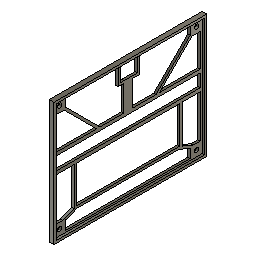
Platine_220 v2 (Autodesk Fusion 360 design; units mm, degrees)
Autodesk Fusion 360 part; units mm, degrees
note: some values were not read from the file. Set by a fixed rule: the direction of a hole.
(part 1 of 10)
sketch "Skizze1" plane through (0, 0, 0) normal (1, 0, 0) x (0, 1, 0)
  line L0 (7.62, 80.01) -> (3.81, 76.2)
  line L1 (99.695, 6.985) -> (99.695, 73.025)
  line L2 (0, 72.39) -> (0, 7.62)
  line L3 (92.71, 80.01) -> (7.62, 80.01)
  line L4 (7.62, 0) -> (92.71, 0)
  line L5 (99.695, 73.025) -> (92.71, 80.01)
  line L6 (3.81, 76.2) -> (0, 72.39)
  line L7 (0, 7.62) -> (7.62, 0)
  line L8 (92.71, 0) -> (99.695, 6.985)
  line L9 (5.5681, 3.81) -> (5.4821, 4.3533)
  line L10 (4.8434, 74.7776) -> (5.2324, 75.1666)
  line L11 (95.9767, 74.5279) -> (96.52, 74.4419)
  line L12 (95.0976, 75.1666) -> (95.4866, 74.7776)
  line L13 (95.9767, 5.4821) -> (95.4866, 5.2324)
  line L14 (5.4821, 4.3533) -> (5.2324, 4.8434)
  line L15 (5.123, 2.6407) -> (5.3653, 2.9903)
  line L16 (97.6893, 74.887) -> (99.5934, 72.9829)
  line L17 (3.3878, 74.4933) -> (3.81, 74.4419)
  line L18 (5.3653, 77.0197) -> (5.123, 77.3693)
  line L19 (94.9647, 77.0197) -> (94.8133, 76.6222)
  line L20 (2.9903, 5.3653) -> (2.6407, 5.123)
  line L21 (99.5934, 7.0271) -> (97.6893, 5.123)
  line L22 (96.52, 74.4419) -> (96.9422, 74.4933)
  line L23 (97.3397, 5.3653) -> (96.9422, 5.5167)
  line L24 (2.6407, 5.123) -> (0.3581, 7.4055)
  line L25 (4.8434, 5.2324) -> (4.3533, 5.4821)
  line L26 (7.4055, 0.3581) -> (5.123, 2.6407)
  line L27 (2.6407, 74.887) -> (2.9903, 74.6447)
  line L28 (0.3581, 7.4055) -> (0.3581, 72.6045)
  line L29 (3.81, 5.5681) -> (3.3878, 5.5167)
  line L30 (94.8133, 76.6222) -> (94.7619, 76.2)
  line L31 (4.3533, 5.4821) -> (3.81, 5.5681)
  line L32 (5.2324, 4.8434) -> (4.8434, 5.2324)
  line L33 (95.4866, 74.7776) -> (95.9767, 74.5279)
  line L34 (97.3397, 74.6447) -> (97.6893, 74.887)
  line L35 (94.8479, 75.6567) -> (95.0976, 75.1666)
  line L36 (94.7619, 3.81) -> (94.8133, 3.3878)
  line L37 (94.9647, 2.9903) -> (95.207, 2.6407)
  line L38 (5.5681, 76.2) -> (5.5167, 76.6222)
  line L39 (2.9903, 74.6447) -> (3.3878, 74.4933)
  line L40 (95.0976, 4.8434) -> (94.8479, 4.3533)
  line L41 (5.4821, 75.6567) -> (5.5681, 76.2)
  line L42 (96.9422, 5.5167) -> (96.52, 5.5681)
  line L43 (94.8133, 3.3878) -> (94.9647, 2.9903)
  line L44 (95.207, 2.6407) -> (92.9245, 0.3581)
  line L45 (94.8479, 4.3533) -> (94.7619, 3.81)
  line L46 (5.123, 77.3693) -> (7.3955, 79.6419)
  line L47 (94.7619, 76.2) -> (94.8479, 75.6567)
  line L48 (92.9245, 0.3581) -> (7.4055, 0.3581)
  line L49 (96.52, 5.5681) -> (95.9767, 5.4821)
  line L50 (97.6893, 5.123) -> (97.3397, 5.3653)
  line L51 (95.4866, 5.2324) -> (95.0976, 4.8434)
  line L52 (99.5934, 72.9829) -> (99.5934, 7.0271)
  line L53 (95.207, 77.3693) -> (94.9647, 77.0197)
  line L54 (4.3533, 74.5279) -> (4.8434, 74.7776)
  line L55 (0.3581, 72.6045) -> (2.6407, 74.887)
  line L56 (3.81, 74.4419) -> (4.3533, 74.5279)
  line L57 (7.3955, 79.6419) -> (92.9345, 79.6419)
  line L58 (5.5167, 76.6222) -> (5.3653, 77.0197)
  line L59 (96.9422, 74.4933) -> (97.3397, 74.6447)
  line L60 (92.9345, 79.6419) -> (95.207, 77.3693)
  line L61 (5.2324, 75.1666) -> (5.4821, 75.6567)
  line L62 (3.3878, 5.5167) -> (2.9903, 5.3653)
  line L63 (5.3653, 2.9903) -> (5.5167, 3.3878)
  line L64 (5.5167, 3.3878) -> (5.5681, 3.81)
  line L65 (66.3187, 30.0127) -> (66.3964, 29.8966)
  line L66 (71.048, 33.3571) -> (71.048, 33.3571)
  line L67 (67.6402, 29.4615) -> (67.6402, 29.4615)
  line L68 (67.6402, 29.4615) -> (67.7773, 29.4887)
  line L69 (72.5965, 32.2321) -> (72.3652, 32.686)
  line L70 (72.5965, 31.2259) -> (72.6761, 31.729)
  line L71 (71.5511, 33.2775) -> (71.048, 33.3571)
  line L72 (66.9595, 32.2321) -> (66.8799, 31.729)
  line L73 (66.8055, 31.4532) -> (66.7266, 31.3936)
  line L74 (68.508, 33.3571) -> (68.508, 33.3571)
  line L75 (66.8799, 31.729) -> (66.8843, 31.6087)
  line L76 (66.7266, 29.5664) -> (66.7266, 29.5664)
  line L77 (66.7266, 31.3936) -> (66.3964, 31.0634)
  line L78 (72.3652, 30.772) -> (72.5965, 31.2259)
  line L79 (66.3964, 31.0634) -> (66.3187, 30.9473)
  line L80 (66.3187, 30.9473) -> (66.2915, 30.8102)
  line L81 (66.3964, 29.8966) -> (66.3964, 29.8966)
  line L82 (66.2915, 30.1498) -> (66.3187, 30.0127)
  line L83 (68.2934, 29.995) -> (68.3264, 30.111)
  line L84 (66.8976, 31.489) -> (66.8055, 31.4532)
  line L85 (72.005, 33.0462) -> (71.5511, 33.2775)
  line L86 (66.8843, 31.6087) -> (66.8976, 31.489)
  line L87 (68.4171, 30.1034) -> (68.508, 30.1009)
  line L88 (66.2915, 30.8102) -> (66.2915, 30.8102)
  line L89 (71.048, 30.1009) -> (71.5511, 30.1805)
  line L90 (72.3652, 32.686) -> (72.005, 33.0462)
  line L91 (67.8934, 29.5664) -> (68.2236, 29.8966)
  line L92 (66.2915, 30.1498) -> (66.2915, 30.1498)
  line L93 (67.8934, 29.5664) -> (67.8934, 29.5664)
  line L94 (68.2236, 29.8966) -> (68.2236, 29.8966)
  line L95 (67.551, 33.0462) -> (67.1908, 32.686)
  line L96 (68.508, 30.1009) -> (68.508, 30.1009)
  line L97 (71.048, 30.1009) -> (71.048, 30.1009)
  line L98 (66.2915, 30.8102) -> (66.2915, 30.1498)
  line L99 (66.3964, 31.0634) -> (66.3964, 31.0634)
  line L100 (68.508, 33.3571) -> (68.0049, 33.2775)
  line L101 (67.1908, 32.686) -> (66.9595, 32.2321)
  line L102 (66.7266, 31.3936) -> (66.7266, 31.3936)
  line L103 (71.048, 33.3571) -> (68.508, 33.3571)
  line L104 (66.7266, 29.5664) -> (66.8427, 29.4887)
  line L105 (71.5511, 30.1805) -> (72.005, 30.4118)
  line L106 (72.005, 30.4118) -> (72.3652, 30.772)
  line L107 (66.3964, 29.8966) -> (66.7266, 29.5664)
  line L108 (67.7773, 29.4887) -> (67.8934, 29.5664)
  line L109 (72.6761, 31.729) -> (72.5965, 32.2321)
  line L110 (66.9798, 29.4615) -> (66.9798, 29.4615)
  line L111 (68.2236, 29.8966) -> (68.2934, 29.995)
  line L112 (66.9798, 29.4615) -> (67.6402, 29.4615)
  line L113 (68.3264, 30.111) -> (68.4171, 30.1034)
  line L114 (66.8427, 29.4887) -> (66.9798, 29.4615)
  line L115 (68.508, 30.1009) -> (71.048, 30.1009)
  line L116 (68.0049, 33.2775) -> (67.551, 33.0462)
  line L117 (92.316, 30.4118) -> (92.7699, 30.1805)
  line L118 (97.4411, 31.729) -> (97.3615, 32.2321)
  line L119 (92.316, 33.0462) -> (91.9558, 32.686)
  line L120 (95.813, 33.3571) -> (95.813, 33.3571)
  line L121 (93.273, 30.1009) -> (95.813, 30.1009)
  line L122 (91.9558, 30.772) -> (92.316, 30.4118)
  line L123 (95.813, 30.1009) -> (95.813, 30.1009)
  line L124 (97.1302, 30.772) -> (97.3615, 31.2259)
  line L125 (92.7699, 33.2775) -> (92.316, 33.0462)
  line L126 (96.3161, 30.1805) -> (96.77, 30.4118)
  line L127 (93.273, 30.1009) -> (93.273, 30.1009)
  line L128 (97.1302, 32.686) -> (96.77, 33.0462)
  line L129 (97.3615, 31.2259) -> (97.4411, 31.729)
  line L130 (93.273, 33.3571) -> (92.7699, 33.2775)
  line L131 (96.77, 30.4118) -> (97.1302, 30.772)
  line L132 (95.813, 30.1009) -> (96.3161, 30.1805)
  line L133 (91.9558, 32.686) -> (91.7245, 32.2321)
  line L134 (93.273, 33.3571) -> (93.273, 33.3571)
  line L135 (96.77, 33.0462) -> (96.3161, 33.2775)
  line L136 (92.7699, 30.1805) -> (93.273, 30.1009)
  line L137 (97.3615, 32.2321) -> (97.1302, 32.686)
  line L138 (95.813, 33.3571) -> (93.273, 33.3571)
  line L139 (91.7245, 31.2259) -> (91.9558, 30.772)
  line L140 (91.6449, 31.729) -> (91.7245, 31.2259)
  line L141 (96.3161, 33.2775) -> (95.813, 33.3571)
  line L142 (91.7245, 32.2321) -> (91.6449, 31.729)
  line L143 (85.3761, 54.729) -> (85.2965, 55.2321)
  line L144 (83.748, 53.1009) -> (84.2511, 53.1805)
  line L145 (85.0652, 53.772) -> (85.2965, 54.2259)
  line L146 (80.251, 56.0462) -> (79.8908, 55.686)
  line L147 (81.208, 56.3571) -> (81.208, 56.3571)
  line L148 (83.748, 53.1009) -> (83.748, 53.1009)
  line L149 (83.748, 56.3571) -> (83.748, 56.3571)
  line L150 (81.208, 53.1009) -> (81.208, 53.1009)
  line L151 (81.208, 53.1009) -> (83.748, 53.1009)
  line L152 (80.251, 53.4118) -> (80.7049, 53.1805)
  line L153 (85.2965, 55.2321) -> (85.0652, 55.686)
  line L154 (84.2511, 53.1805) -> (84.705, 53.4118)
  line L155 (85.0652, 55.686) -> (84.705, 56.0462)
  line L156 (81.208, 56.3571) -> (80.7049, 56.2775)
  line L157 (80.7049, 53.1805) -> (81.208, 53.1009)
  line L158 (79.6595, 55.2321) -> (79.5799, 54.729)
  line L159 (84.2511, 56.2775) -> (83.748, 56.3571)
  line L160 (84.705, 53.4118) -> (85.0652, 53.772)
  line L161 (79.8908, 53.772) -> (80.251, 53.4118)
  line L162 (83.748, 56.3571) -> (81.208, 56.3571)
  line L163 (80.7049, 56.2775) -> (80.251, 56.0462)
  line L164 (79.8908, 55.686) -> (79.6595, 55.2321)
  line L165 (85.2965, 54.2259) -> (85.3761, 54.729)
  line L166 (84.705, 56.0462) -> (84.2511, 56.2775)
  line L167 (79.5799, 54.729) -> (79.6595, 54.2259)
  line L168 (79.6595, 54.2259) -> (79.8908, 53.772)
  line L169 (91.6449, 54.729) -> (91.7245, 54.2259)
  line L170 (93.273, 53.1009) -> (93.273, 53.1009)
  line L171 (91.9558, 53.772) -> (92.316, 53.4118)
  line L172 (96.77, 53.4118) -> (97.1302, 53.772)
  line L173 (91.7245, 54.2259) -> (91.9558, 53.772)
  line L174 (93.273, 56.3571) -> (92.7699, 56.2775)
  line L175 (96.77, 56.0462) -> (96.3161, 56.2775)
  line L176 (96.3161, 56.2775) -> (95.813, 56.3571)
  line L177 (92.316, 56.0462) -> (91.9558, 55.686)
  line L178 (96.3161, 53.1805) -> (96.77, 53.4118)
  line L179 (95.813, 56.3571) -> (93.273, 56.3571)
  line L180 (97.1302, 55.686) -> (96.77, 56.0462)
  line L181 (97.4411, 54.729) -> (97.3615, 55.2321)
  line L182 (95.813, 56.3571) -> (95.813, 56.3571)
  line L183 (95.813, 53.1009) -> (95.813, 53.1009)
  line L184 (92.7699, 56.2775) -> (92.316, 56.0462)
  line L185 (92.7699, 53.1805) -> (93.273, 53.1009)
  line L186 (93.273, 53.1009) -> (95.813, 53.1009)
  line L187 (91.9558, 55.686) -> (91.7245, 55.2321)
  line L188 (97.1302, 53.772) -> (97.3615, 54.2259)
  line L189 (91.7245, 55.2321) -> (91.6449, 54.729)
  line L190 (95.813, 53.1009) -> (96.3161, 53.1805)
  line L191 (97.3615, 55.2321) -> (97.1302, 55.686)
  line L192 (97.3615, 54.2259) -> (97.4411, 54.729)
  line L193 (92.316, 53.4118) -> (92.7699, 53.1805)
  line L194 (93.273, 56.3571) -> (93.273, 56.3571)
  line L195 (72.005, 56.0462) -> (71.5511, 56.2775)
  line L196 (66.8799, 54.729) -> (66.9595, 54.2259)
  line L197 (68.508, 56.3571) -> (68.508, 56.3571)
  line L198 (71.048, 53.1009) -> (71.048, 53.1009)
  line L199 (66.9595, 54.2259) -> (67.1908, 53.772)
  line L200 (72.005, 53.4118) -> (72.3652, 53.772)
  line L201 (68.508, 53.1009) -> (68.508, 53.1009)
  line L202 (67.1908, 55.686) -> (66.9595, 55.2321)
  line L203 (71.048, 56.3571) -> (68.508, 56.3571)
  line L204 (68.0049, 53.1805) -> (68.508, 53.1009)
  line L205 (71.5511, 56.2775) -> (71.048, 56.3571)
  line L206 (71.048, 53.1009) -> (71.5511, 53.1805)
  line L207 (67.551, 56.0462) -> (67.1908, 55.686)
  line L208 (72.3652, 53.772) -> (72.5965, 54.2259)
  line L209 (68.508, 53.1009) -> (71.048, 53.1009)
  line L210 (67.551, 53.4118) -> (68.0049, 53.1805)
  line L211 (68.0049, 56.2775) -> (67.551, 56.0462)
  line L212 (67.1908, 53.772) -> (67.551, 53.4118)
  line L213 (72.3652, 55.686) -> (72.005, 56.0462)
  line L214 (72.5965, 55.2321) -> (72.3652, 55.686)
  line L215 (72.5965, 54.2259) -> (72.6761, 54.729)
  line L216 (72.6761, 54.729) -> (72.5965, 55.2321)
  line L217 (66.9595, 55.2321) -> (66.8799, 54.729)
  line L218 (68.508, 56.3571) -> (68.0049, 56.2775)
  line L219 (71.048, 56.3571) -> (71.048, 56.3571)
  line L220 (71.5511, 53.1805) -> (72.005, 53.4118)
  line L221 (83.748, 33.3571) -> (83.748, 33.3571)
  line L222 (80.7049, 30.1805) -> (81.208, 30.1009)
  line L223 (79.6595, 31.2259) -> (79.8908, 30.772)
  line L224 (81.208, 33.3571) -> (81.208, 33.3571)
  line L225 (85.0652, 30.772) -> (85.2965, 31.2259)
  line L226 (80.251, 33.0462) -> (79.8908, 32.686)
  line L227 (84.2511, 33.2775) -> (83.748, 33.3571)
  line L228 (85.3761, 31.729) -> (85.2965, 32.2321)
  line L229 (83.748, 30.1009) -> (83.748, 30.1009)
  line L230 (84.2511, 30.1805) -> (84.705, 30.4118)
  line L231 (80.7049, 33.2775) -> (80.251, 33.0462)
  line L232 (80.251, 30.4118) -> (80.7049, 30.1805)
  line L233 (85.2965, 31.2259) -> (85.3761, 31.729)
  line L234 (81.208, 30.1009) -> (81.208, 30.1009)
  line L235 (85.0652, 32.686) -> (84.705, 33.0462)
  line L236 (79.8908, 32.686) -> (79.6595, 32.2321)
  line L237 (79.5799, 31.729) -> (79.6595, 31.2259)
  line L238 (81.208, 30.1009) -> (83.748, 30.1009)
  line L239 (79.6595, 32.2321) -> (79.5799, 31.729)
  line L240 (84.705, 30.4118) -> (85.0652, 30.772)
  line L241 (81.208, 33.3571) -> (80.7049, 33.2775)
  line L242 (85.2965, 32.2321) -> (85.0652, 32.686)
  line L243 (79.8908, 30.772) -> (80.251, 30.4118)
  line L244 (84.705, 33.0462) -> (84.2511, 33.2775)
  line L245 (83.748, 33.3571) -> (81.208, 33.3571)
  line L246 (83.748, 30.1009) -> (84.2511, 30.1805)
  line L247 (6.913, 53.1009) -> (7.4161, 53.1805)
  line L248 (4.373, 53.1009) -> (6.913, 53.1009)
  line L249 (6.913, 53.1009) -> (6.913, 53.1009)
  line L250 (2.7449, 54.729) -> (2.8245, 54.2259)
  line L251 (3.416, 56.0462) -> (3.0558, 55.686)
  line L252 (2.8245, 55.2321) -> (2.7449, 54.729)
  line L253 (7.87, 53.4118) -> (8.2302, 53.772)
  line L254 (6.913, 56.3571) -> (6.913, 56.3571)
  line L255 (7.4161, 53.1805) -> (7.87, 53.4118)
  line L256 (3.0558, 55.686) -> (2.8245, 55.2321)
  line L257 (6.913, 56.3571) -> (4.373, 56.3571)
  line L258 (8.5411, 54.729) -> (8.4615, 55.2321)
  line L259 (3.8699, 56.2775) -> (3.416, 56.0462)
  line L260 (3.0558, 53.772) -> (3.416, 53.4118)
  line L261 (3.8699, 53.1805) -> (4.373, 53.1009)
  line L262 (7.87, 56.0462) -> (7.4161, 56.2775)
  line L263 (3.416, 53.4118) -> (3.8699, 53.1805)
  line L264 (2.8245, 54.2259) -> (3.0558, 53.772)
  line L265 (4.373, 53.1009) -> (4.373, 53.1009)
  line L266 (8.4615, 54.2259) -> (8.5411, 54.729)
  line L267 (8.2302, 53.772) -> (8.4615, 54.2259)
  line L268 (4.373, 56.3571) -> (3.8699, 56.2775)
  line L269 (4.373, 56.3571) -> (4.373, 56.3571)
  line L270 (8.4615, 55.2321) -> (8.2302, 55.686)
  line L271 (7.4161, 56.2775) -> (6.913, 56.3571)
  line L272 (8.2302, 55.686) -> (7.87, 56.0462)
  line L273 (28.2245, 54.2259) -> (28.4558, 53.772)
  line L274 (28.816, 56.0462) -> (28.4558, 55.686)
  line L275 (28.816, 53.4118) -> (29.2699, 53.1805)
  line L276 (33.27, 56.0462) -> (32.8161, 56.2775)
  line L277 (32.313, 56.3571) -> (32.313, 56.3571)
  line L278 (33.6302, 53.772) -> (33.8615, 54.2259)
  line L279 (33.8615, 55.2321) -> (33.6302, 55.686)
  line L280 (33.9411, 54.729) -> (33.8615, 55.2321)
  line L281 (29.773, 53.1009) -> (29.773, 53.1009)
  line L282 (29.2699, 53.1805) -> (29.773, 53.1009)
  line L283 (32.313, 53.1009) -> (32.8161, 53.1805)
  line L284 (28.4558, 55.686) -> (28.2245, 55.2321)
  line L285 (32.313, 56.3571) -> (29.773, 56.3571)
  line L286 (28.2245, 55.2321) -> (28.1449, 54.729)
  line L287 (33.27, 53.4118) -> (33.6302, 53.772)
  line L288 (32.313, 53.1009) -> (32.313, 53.1009)
  line L289 (33.8615, 54.2259) -> (33.9411, 54.729)
  line L290 (29.773, 56.3571) -> (29.2699, 56.2775)
  line L291 (29.2699, 56.2775) -> (28.816, 56.0462)
  line L292 (33.6302, 55.686) -> (33.27, 56.0462)
  line L293 (28.1449, 54.729) -> (28.2245, 54.2259)
  line L294 (29.773, 56.3571) -> (29.773, 56.3571)
  line L295 (32.8161, 56.2775) -> (32.313, 56.3571)
  line L296 (32.8161, 53.1805) -> (33.27, 53.4118)
  line L297 (28.4558, 53.772) -> (28.816, 53.4118)
  line L298 (29.773, 53.1009) -> (32.313, 53.1009)
  line L299 (1.8919, 65.99) -> (1.8919, 65.99)
  line L300 (2.563, 62.1328) -> (3.0169, 61.9015)
  line L301 (4.477, 67.3072) -> (4.0231, 67.5385)
  line L302 (4.8372, 62.493) -> (5.0685, 62.9469)
  line L303 (2.2028, 66.947) -> (1.9715, 66.4931)
  line L304 (5.1481, 63.45) -> (5.1481, 65.99)
  line L305 (5.0685, 66.4931) -> (4.8372, 66.947)
  line L306 (5.1481, 65.99) -> (5.1481, 65.99)
  line L307 (1.8919, 65.99) -> (1.8919, 63.45)
  line L308 (3.52, 67.6181) -> (3.0169, 67.5385)
  line L309 (4.8372, 66.947) -> (4.477, 67.3072)
  line L310 (1.8919, 63.45) -> (1.9715, 62.9469)
  line L311 (2.2028, 62.493) -> (2.563, 62.1328)
  line L312 (5.1481, 65.99) -> (5.0685, 66.4931)
  line L313 (3.0169, 61.9015) -> (3.52, 61.8219)
  line L314 (3.52, 61.8219) -> (4.0231, 61.9015)
  line L315 (4.0231, 61.9015) -> (4.477, 62.1328)
  line L316 (4.477, 62.1328) -> (4.8372, 62.493)
  line L317 (1.9715, 66.4931) -> (1.8919, 65.99)
  line L318 (2.563, 67.3072) -> (2.2028, 66.947)
  line L319 (5.1481, 63.45) -> (5.1481, 63.45)
  line L320 (1.8919, 63.45) -> (1.8919, 63.45)
  line L321 (5.0685, 62.9469) -> (5.1481, 63.45)
  line L322 (3.0169, 67.5385) -> (2.563, 67.3072)
  line L323 (4.0231, 67.5385) -> (3.52, 67.6181)
  line L324 (1.9715, 62.9469) -> (2.2028, 62.493)
  line L325 (98.4381, 63.55) -> (98.4381, 63.55)
  line L326 (96.3069, 62.0015) -> (96.81, 61.9219)
  line L327 (98.4381, 66.09) -> (98.3585, 66.5931)
  line L328 (97.767, 62.2328) -> (98.1272, 62.593)
  line L329 (98.1272, 62.593) -> (98.3585, 63.0469)
  line L330 (98.4381, 63.55) -> (98.4381, 66.09)
  line L331 (95.1819, 63.55) -> (95.2615, 63.0469)
  line L332 (98.3585, 63.0469) -> (98.4381, 63.55)
  line L333 (97.3131, 62.0015) -> (97.767, 62.2328)
  line L334 (95.1819, 66.09) -> (95.1819, 63.55)
  line L335 (95.1819, 63.55) -> (95.1819, 63.55)
  line L336 (96.3069, 67.6385) -> (95.853, 67.4072)
  line L337 (95.2615, 66.5931) -> (95.1819, 66.09)
  line L338 (98.1272, 67.047) -> (97.767, 67.4072)
  line L339 (98.3585, 66.5931) -> (98.1272, 67.047)
  line L340 (95.4928, 67.047) -> (95.2615, 66.5931)
  line L341 (97.767, 67.4072) -> (97.3131, 67.6385)
  line L342 (95.853, 62.2328) -> (96.3069, 62.0015)
  line L343 (96.81, 67.7181) -> (96.3069, 67.6385)
  line L344 (96.81, 61.9219) -> (97.3131, 62.0015)
  line L345 (95.853, 67.4072) -> (95.4928, 67.047)
  line L346 (95.2615, 63.0469) -> (95.4928, 62.593)
  line L347 (98.4381, 66.09) -> (98.4381, 66.09)
  line L348 (95.4928, 62.593) -> (95.853, 62.2328)
  line L349 (95.1819, 66.09) -> (95.1819, 66.09)
  line L350 (97.3131, 67.6385) -> (96.81, 67.7181)
  line L351 (17.073, 56.3571) -> (17.073, 56.3571)
  line L352 (16.116, 56.0462) -> (15.7558, 55.686)
  line L353 (20.57, 56.0462) -> (20.1161, 56.2775)
  line L354 (16.5699, 56.2775) -> (16.116, 56.0462)
  line L355 (16.5699, 53.1805) -> (17.073, 53.1009)
  line L356 (15.7558, 53.772) -> (16.116, 53.4118)
  line L357 (16.116, 53.4118) -> (16.5699, 53.1805)
  line L358 (19.613, 56.3571) -> (19.613, 56.3571)
  line L359 (17.073, 53.1009) -> (17.073, 53.1009)
  line L360 (17.073, 56.3571) -> (16.5699, 56.2775)
  line L361 (15.4449, 54.729) -> (15.5245, 54.2259)
  line L362 (17.073, 53.1009) -> (19.613, 53.1009)
  line L363 (19.613, 53.1009) -> (19.613, 53.1009)
  line L364 (20.1161, 56.2775) -> (19.613, 56.3571)
  line L365 (21.1615, 55.2321) -> (20.9302, 55.686)
  line L366 (21.1615, 54.2259) -> (21.2411, 54.729)
  line L367 (19.613, 56.3571) -> (17.073, 56.3571)
  line L368 (20.9302, 55.686) -> (20.57, 56.0462)
  line L369 (21.2411, 54.729) -> (21.1615, 55.2321)
  line L370 (19.613, 53.1009) -> (20.1161, 53.1805)
  line L371 (20.57, 53.4118) -> (20.9302, 53.772)
  line L372 (15.5245, 55.2321) -> (15.4449, 54.729)
  line L373 (20.9302, 53.772) -> (21.1615, 54.2259)
  line L374 (15.7558, 55.686) -> (15.5245, 55.2321)
  line L375 (15.5245, 54.2259) -> (15.7558, 53.772)
  line L376 (20.1161, 53.1805) -> (20.57, 53.4118)
  line L377 (58.348, 56.3571) -> (55.808, 56.3571)
  line L378 (59.305, 53.4118) -> (59.6652, 53.772)
  line L379 (54.1799, 54.729) -> (54.2595, 54.2259)
  line L380 (58.348, 53.1009) -> (58.348, 53.1009)
  line L381 (55.808, 56.3571) -> (55.3049, 56.2775)
  line L382 (54.2595, 54.2259) -> (54.4908, 53.772)
  line L383 (59.8965, 54.2259) -> (59.9761, 54.729)
  line L384 (58.348, 53.1009) -> (58.8511, 53.1805)
  line L385 (55.808, 53.1009) -> (55.808, 53.1009)
  line L386 (59.6652, 53.772) -> (59.8965, 54.2259)
  line L387 (54.4908, 55.686) -> (54.2595, 55.2321)
  line L388 (54.851, 56.0462) -> (54.4908, 55.686)
  line L389 (55.3049, 56.2775) -> (54.851, 56.0462)
  line L390 (59.9761, 54.729) -> (59.8965, 55.2321)
  line L391 (54.851, 53.4118) -> (55.3049, 53.1805)
  line L392 (55.3049, 53.1805) -> (55.808, 53.1009)
  line L393 (59.305, 56.0462) -> (58.8511, 56.2775)
  line L394 (54.4908, 53.772) -> (54.851, 53.4118)
  line L395 (55.808, 53.1009) -> (58.348, 53.1009)
  line L396 (58.348, 56.3571) -> (58.348, 56.3571)
  line L397 (58.8511, 56.2775) -> (58.348, 56.3571)
  line L398 (59.6652, 55.686) -> (59.305, 56.0462)
  line L399 (59.8965, 55.2321) -> (59.6652, 55.686)
  line L400 (58.8511, 53.1805) -> (59.305, 53.4118)
  line L401 (55.808, 56.3571) -> (55.808, 56.3571)
  line L402 (54.2595, 55.2321) -> (54.1799, 54.729)
  line L403 (42.473, 56.3571) -> (42.473, 56.3571)
  line L404 (41.1558, 55.686) -> (40.9245, 55.2321)
  line L405 (45.5161, 53.1805) -> (45.97, 53.4118)
  line L406 (46.5615, 55.2321) -> (46.3302, 55.686)
  line L407 (46.3302, 53.772) -> (46.5615, 54.2259)
  line L408 (41.516, 56.0462) -> (41.1558, 55.686)
  line L409 (40.8449, 54.729) -> (40.9245, 54.2259)
  line L410 (42.473, 53.1009) -> (45.013, 53.1009)
  line L411 (41.516, 53.4118) -> (41.9699, 53.1805)
  line L412 (45.013, 53.1009) -> (45.013, 53.1009)
  line L413 (40.9245, 54.2259) -> (41.1558, 53.772)
  line L414 (41.1558, 53.772) -> (41.516, 53.4118)
  line L415 (41.9699, 53.1805) -> (42.473, 53.1009)
  line L416 (41.9699, 56.2775) -> (41.516, 56.0462)
  line L417 (45.013, 56.3571) -> (45.013, 56.3571)
  line L418 (45.5161, 56.2775) -> (45.013, 56.3571)
  line L419 (45.97, 53.4118) -> (46.3302, 53.772)
  line L420 (46.5615, 54.2259) -> (46.6411, 54.729)
  line L421 (42.473, 56.3571) -> (41.9699, 56.2775)
  line L422 (46.3302, 55.686) -> (45.97, 56.0462)
  line L423 (40.9245, 55.2321) -> (40.8449, 54.729)
  line L424 (45.013, 56.3571) -> (42.473, 56.3571)
  line L425 (42.473, 53.1009) -> (42.473, 53.1009)
  line L426 (45.013, 53.1009) -> (45.5161, 53.1805)
  line L427 (46.6411, 54.729) -> (46.5615, 55.2321)
  line L428 (45.97, 56.0462) -> (45.5161, 56.2775)
  line L429 (28.1449, 31.729) -> (28.2245, 31.2259)
  line L430 (33.9411, 31.729) -> (33.8615, 32.2321)
  line L431 (32.8161, 33.2775) -> (32.313, 33.3571)
  line L432 (32.8161, 30.1805) -> (33.27, 30.4118)
  line L433 (29.2699, 33.2775) -> (28.816, 33.0462)
  line L434 (28.2245, 31.2259) -> (28.4558, 30.772)
  line L435 (33.6302, 30.772) -> (33.8615, 31.2259)
  line L436 (32.313, 33.3571) -> (29.773, 33.3571)
  line L437 (28.816, 33.0462) -> (28.4558, 32.686)
  line L438 (29.773, 30.1009) -> (32.313, 30.1009)
  line L439 (32.313, 30.1009) -> (32.8161, 30.1805)
  line L440 (32.313, 30.1009) -> (32.313, 30.1009)
  line L441 (29.2699, 30.1805) -> (29.773, 30.1009)
  line L442 (33.27, 33.0462) -> (32.8161, 33.2775)
  line L443 (33.27, 30.4118) -> (33.6302, 30.772)
  line L444 (29.773, 33.3571) -> (29.773, 33.3571)
  line L445 (28.2245, 32.2321) -> (28.1449, 31.729)
  line L446 (33.8615, 31.2259) -> (33.9411, 31.729)
  line L447 (32.313, 33.3571) -> (32.313, 33.3571)
  line L448 (28.4558, 32.686) -> (28.2245, 32.2321)
  line L449 (28.4558, 30.772) -> (28.816, 30.4118)
  line L450 (33.6302, 32.686) -> (33.27, 33.0462)
  line L451 (33.8615, 32.2321) -> (33.6302, 32.686)
  line L452 (29.773, 30.1009) -> (29.773, 30.1009)
  line L453 (29.773, 33.3571) -> (29.2699, 33.2775)
  line L454 (28.816, 30.4118) -> (29.2699, 30.1805)
  line L455 (21.2411, 31.729) -> (21.1615, 32.2321)
  line L456 (19.613, 33.3571) -> (19.613, 33.3571)
  line L457 (20.9302, 32.686) -> (20.57, 33.0462)
  line L458 (17.073, 33.3571) -> (17.073, 33.3571)
  line L459 (20.57, 30.4118) -> (20.9302, 30.772)
  line L460 (17.073, 33.3571) -> (16.5699, 33.2775)
  line L461 (20.9302, 30.772) -> (21.1615, 31.2259)
  line L462 (16.5699, 33.2775) -> (16.116, 33.0462)
  line L463 (20.57, 33.0462) -> (20.1161, 33.2775)
  line L464 (20.1161, 30.1805) -> (20.57, 30.4118)
  line L465 (19.613, 30.1009) -> (20.1161, 30.1805)
  line L466 (20.1161, 33.2775) -> (19.613, 33.3571)
  line L467 (15.5245, 31.2259) -> (15.7558, 30.772)
  line L468 (17.073, 30.1009) -> (17.073, 30.1009)
  line L469 (15.7558, 32.686) -> (15.5245, 32.2321)
  line L470 (16.5699, 30.1805) -> (17.073, 30.1009)
  line L471 (19.613, 30.1009) -> (19.613, 30.1009)
  line L472 (15.5245, 32.2321) -> (15.4449, 31.729)
  line L473 (21.1615, 31.2259) -> (21.2411, 31.729)
  line L474 (17.073, 30.1009) -> (19.613, 30.1009)
  line L475 (16.116, 30.4118) -> (16.5699, 30.1805)
  line L476 (19.613, 33.3571) -> (17.073, 33.3571)
  line L477 (21.1615, 32.2321) -> (20.9302, 32.686)
  line L478 (15.4449, 31.729) -> (15.5245, 31.2259)
  line L479 (16.116, 33.0462) -> (15.7558, 32.686)
  line L480 (15.7558, 30.772) -> (16.116, 30.4118)
  line L481 (54.4908, 30.772) -> (54.851, 30.4118)
  line L482 (55.808, 30.1009) -> (55.808, 30.1009)
  line L483 (54.1799, 31.729) -> (54.2595, 31.2259)
  line L484 (59.8965, 32.2321) -> (59.6652, 32.686)
  line L485 (54.851, 30.4118) -> (55.3049, 30.1805)
  line L486 (58.348, 30.1009) -> (58.348, 30.1009)
  line L487 (59.6652, 30.772) -> (59.8965, 31.2259)
  line L488 (54.2595, 31.2259) -> (54.4908, 30.772)
  line L489 (54.851, 33.0462) -> (54.4908, 32.686)
  line L490 (54.4908, 32.686) -> (54.2595, 32.2321)
  line L491 (59.305, 30.4118) -> (59.6652, 30.772)
  line L492 (58.8511, 33.2775) -> (58.348, 33.3571)
  line L493 (55.808, 30.1009) -> (58.348, 30.1009)
  line L494 (54.2595, 32.2321) -> (54.1799, 31.729)
  line L495 (55.3049, 30.1805) -> (55.808, 30.1009)
  line L496 (55.808, 33.3571) -> (55.3049, 33.2775)
  line L497 (58.348, 33.3571) -> (58.348, 33.3571)
  line L498 (59.9761, 31.729) -> (59.8965, 32.2321)
  line L499 (58.8511, 30.1805) -> (59.305, 30.4118)
  line L500 (59.305, 33.0462) -> (58.8511, 33.2775)
  line L501 (59.6652, 32.686) -> (59.305, 33.0462)
  line L502 (58.348, 33.3571) -> (55.808, 33.3571)
  line L503 (59.8965, 31.2259) -> (59.9761, 31.729)
  line L504 (55.3049, 33.2775) -> (54.851, 33.0462)
  line L505 (58.348, 30.1009) -> (58.8511, 30.1805)
  line L506 (55.808, 33.3571) -> (55.808, 33.3571)
  line L507 (42.473, 30.1009) -> (45.013, 30.1009)
  line L508 (40.9245, 31.2259) -> (41.1558, 30.772)
  line L509 (45.013, 33.3571) -> (45.013, 33.3571)
  line L510 (45.5161, 30.1805) -> (45.97, 30.4118)
  line L511 (40.8449, 31.729) -> (40.9245, 31.2259)
  line L512 (42.473, 30.1009) -> (42.473, 30.1009)
  line L513 (41.1558, 30.772) -> (41.516, 30.4118)
  line L514 (41.9699, 30.1805) -> (42.473, 30.1009)
  line L515 (46.5615, 31.2259) -> (46.6411, 31.729)
  line L516 (46.3302, 32.686) -> (45.97, 33.0462)
  line L517 (45.97, 30.4118) -> (46.3302, 30.772)
  line L518 (46.6411, 31.729) -> (46.5615, 32.2321)
  line L519 (45.013, 30.1009) -> (45.5161, 30.1805)
  line L520 (41.516, 30.4118) -> (41.9699, 30.1805)
  line L521 (46.5615, 32.2321) -> (46.3302, 32.686)
  line L522 (41.516, 33.0462) -> (41.1558, 32.686)
  line L523 (42.473, 33.3571) -> (41.9699, 33.2775)
  line L524 (41.1558, 32.686) -> (40.9245, 32.2321)
  line L525 (46.3302, 30.772) -> (46.5615, 31.2259)
  line L526 (45.97, 33.0462) -> (45.5161, 33.2775)
  line L527 (42.473, 33.3571) -> (42.473, 33.3571)
  line L528 (45.013, 30.1009) -> (45.013, 30.1009)
  line L529 (41.9699, 33.2775) -> (41.516, 33.0462)
  line L530 (45.5161, 33.2775) -> (45.013, 33.3571)
  line L531 (45.013, 33.3571) -> (42.473, 33.3571)
  line L532 (40.9245, 32.2321) -> (40.8449, 31.729)
  line L533 (37.02, 67.5931) -> (36.5169, 67.5135)
  line L534 (36.063, 62.1078) -> (36.5169, 61.8765)
  line L535 (37.977, 62.1078) -> (38.3372, 62.468)
  line L536 (38.5685, 62.9219) -> (38.6481, 63.425)
  line L537 (35.3919, 63.425) -> (35.3919, 63.425)
  line L538 (38.5685, 66.4681) -> (38.3372, 66.922)
  line L539 (37.5231, 61.8765) -> (37.977, 62.1078)
  line L540 (38.3372, 66.922) -> (37.977, 67.2822)
  line L541 (35.7028, 62.468) -> (36.063, 62.1078)
  line L542 (35.4715, 66.4681) -> (35.3919, 65.965)
  line L543 (37.5231, 67.5135) -> (37.02, 67.5931)
  line L544 (35.7028, 66.922) -> (35.4715, 66.4681)
  line L545 (36.5169, 61.8765) -> (37.02, 61.7969)
  line L546 (38.3372, 62.468) -> (38.5685, 62.9219)
  line L547 (36.063, 67.2822) -> (35.7028, 66.922)
  line L548 (35.3919, 65.965) -> (35.3919, 65.965)
  line L549 (37.02, 61.7969) -> (37.5231, 61.8765)
  line L550 (36.5169, 67.5135) -> (36.063, 67.2822)
  line L551 (38.6481, 63.425) -> (38.6481, 65.965)
  line L552 (38.6481, 63.425) -> (38.6481, 63.425)
  line L553 (38.6481, 65.965) -> (38.6481, 65.965)
  line L554 (35.3919, 65.965) -> (35.3919, 63.425)
  line L555 (35.4715, 62.9219) -> (35.7028, 62.468)
  line L556 (38.6481, 65.965) -> (38.5685, 66.4681)
  line L557 (35.3919, 63.425) -> (35.4715, 62.9219)
  line L558 (37.977, 67.2822) -> (37.5231, 67.5135)
  line L559 (3.8699, 33.2775) -> (3.416, 33.0462)
  line L560 (2.7449, 31.729) -> (2.8245, 31.2259)
  line L561 (8.5411, 31.729) -> (8.4615, 32.2321)
  line L562 (8.2302, 32.686) -> (7.87, 33.0462)
  line L563 (2.8245, 31.2259) -> (3.0558, 30.772)
  line L564 (3.8699, 30.1805) -> (4.373, 30.1009)
  line L565 (3.0558, 32.686) -> (2.8245, 32.2321)
  line L566 (4.373, 30.1009) -> (4.373, 30.1009)
  line L567 (2.8245, 32.2321) -> (2.7449, 31.729)
  line L568 (8.4615, 32.2321) -> (8.2302, 32.686)
  line L569 (7.87, 33.0462) -> (7.4161, 33.2775)
  line L570 (7.4161, 33.2775) -> (6.913, 33.3571)
  line L571 (7.4161, 30.1805) -> (7.87, 30.4118)
  line L572 (6.913, 30.1009) -> (6.913, 30.1009)
  line L573 (6.913, 33.3571) -> (4.373, 33.3571)
  line L574 (6.913, 30.1009) -> (7.4161, 30.1805)
  line L575 (4.373, 33.3571) -> (4.373, 33.3571)
  line L576 (3.416, 30.4118) -> (3.8699, 30.1805)
  line L577 (4.373, 30.1009) -> (6.913, 30.1009)
  line L578 (6.913, 33.3571) -> (6.913, 33.3571)
  line L579 (7.87, 30.4118) -> (8.2302, 30.772)
  line L580 (8.4615, 31.2259) -> (8.5411, 31.729)
  line L581 (4.373, 33.3571) -> (3.8699, 33.2775)
  line L582 (3.0558, 30.772) -> (3.416, 30.4118)
  line L583 (3.416, 33.0462) -> (3.0558, 32.686)
  line L584 (8.2302, 30.772) -> (8.4615, 31.2259)
  line L585 (61.6819, 66.115) -> (61.6819, 63.575)
  line L586 (61.6819, 63.575) -> (61.6819, 63.575)
  line L587 (64.8585, 66.6181) -> (64.6272, 67.072)
  line L588 (64.6272, 62.618) -> (64.8585, 63.0719)
  line L589 (64.6272, 67.072) -> (64.267, 67.4322)
  line L590 (62.8069, 62.0265) -> (63.31, 61.9469)
  line L591 (61.6819, 63.575) -> (61.7615, 63.0719)
  line L592 (62.353, 67.4322) -> (61.9928, 67.072)
  line L593 (61.7615, 66.6181) -> (61.6819, 66.115)
  line L594 (63.8131, 62.0265) -> (64.267, 62.2578)
  line L595 (61.9928, 62.618) -> (62.353, 62.2578)
  line L596 (62.353, 62.2578) -> (62.8069, 62.0265)
  line L597 (61.7615, 63.0719) -> (61.9928, 62.618)
  line L598 (64.267, 62.2578) -> (64.6272, 62.618)
  line L599 (64.9381, 63.575) -> (64.9381, 63.575)
  line L600 (61.6819, 66.115) -> (61.6819, 66.115)
  line L601 (62.8069, 67.6635) -> (62.353, 67.4322)
  line L602 (63.31, 67.7431) -> (62.8069, 67.6635)
  line L603 (64.9381, 66.115) -> (64.8585, 66.6181)
  line L604 (61.9928, 67.072) -> (61.7615, 66.6181)
  line L605 (63.8131, 67.6635) -> (63.31, 67.7431)
  line L606 (64.9381, 66.115) -> (64.9381, 66.115)
  line L607 (64.9381, 63.575) -> (64.9381, 66.115)
  line L608 (64.8585, 63.0719) -> (64.9381, 63.575)
  line L609 (64.267, 67.4322) -> (63.8131, 67.6635)
  line L610 (63.31, 61.9469) -> (63.8131, 62.0265)
  line L611 (48.6951, 77.7642) -> (48.26, 77.8331)
  line L612 (47.4323, 73.1858) -> (47.8249, 72.9858)
  line L613 (47.4323, 77.5642) -> (47.1208, 77.2527)
  line L614 (48.26, 77.8331) -> (47.8249, 77.7642)
  line L615 (46.8519, 76.425) -> (46.8519, 74.325)
  line L616 (47.8249, 72.9858) -> (48.26, 72.9169)
  line L617 (46.8519, 74.325) -> (46.8519, 74.325)
  line L618 (49.6681, 76.425) -> (49.5992, 76.8601)
  line L619 (46.8519, 74.325) -> (46.9208, 73.8899)
  line L620 (47.8249, 77.7642) -> (47.4323, 77.5642)
  line L621 (49.6681, 76.425) -> (49.6681, 76.425)
  line L622 (49.3992, 73.4973) -> (49.5992, 73.8899)
  line L623 (49.3992, 77.2527) -> (49.0877, 77.5642)
  line L624 (49.5992, 76.8601) -> (49.3992, 77.2527)
  line L625 (47.1208, 73.4973) -> (47.4323, 73.1858)
  line L626 (49.5992, 73.8899) -> (49.6681, 74.325)
  line L627 (49.6681, 74.325) -> (49.6681, 74.325)
  line L628 (48.26, 72.9169) -> (48.6951, 72.9858)
  line L629 (49.6681, 74.325) -> (49.6681, 76.425)
  line L630 (48.6951, 72.9858) -> (49.0877, 73.1858)
  line L631 (49.0877, 77.5642) -> (48.6951, 77.7642)
  line L632 (49.0877, 73.1858) -> (49.3992, 73.4973)
  line L633 (46.9208, 76.8601) -> (46.8519, 76.425)
  line L634 (47.1208, 77.2527) -> (46.9208, 76.8601)
  line L635 (46.8519, 76.425) -> (46.8519, 76.425)
  line L636 (46.9208, 73.8899) -> (47.1208, 73.4973)
  line L637 (94.39, 17.2831) -> (93.9549, 17.2142)
  line L638 (93.9549, 14.5358) -> (94.39, 14.4669)
  line L639 (96.49, 17.2831) -> (96.49, 17.2831)
  line L640 (93.2508, 16.7027) -> (93.0508, 16.3101)
  line L641 (93.0508, 15.4399) -> (93.2508, 15.0473)
  line L642 (97.8981, 15.875) -> (97.8292, 16.3101)
  line L643 (97.8292, 16.3101) -> (97.6292, 16.7027)
  line L644 (97.6292, 16.7027) -> (97.3177, 17.0142)
  line L645 (94.39, 14.4669) -> (94.39, 14.4669)
  line L646 (93.2508, 15.0473) -> (93.5623, 14.7358)
  line L647 (96.49, 14.4669) -> (96.49, 14.4669)
  line L648 (93.5623, 14.7358) -> (93.9549, 14.5358)
  line L649 (93.0508, 16.3101) -> (92.9819, 15.875)
  line L650 (93.9549, 17.2142) -> (93.5623, 17.0142)
  line L651 (97.3177, 14.7358) -> (97.6292, 15.0473)
  line L652 (97.6292, 15.0473) -> (97.8292, 15.4399)
  line L653 (97.8292, 15.4399) -> (97.8981, 15.875)
  line L654 (96.49, 14.4669) -> (96.9251, 14.5358)
  line L655 (96.49, 17.2831) -> (94.39, 17.2831)
  line L656 (94.39, 14.4669) -> (96.49, 14.4669)
  line L657 (96.9251, 17.2142) -> (96.49, 17.2831)
  line L658 (96.9251, 14.5358) -> (97.3177, 14.7358)
  line L659 (94.39, 17.2831) -> (94.39, 17.2831)
  line L660 (97.3177, 17.0142) -> (96.9251, 17.2142)
  line L661 (92.9819, 15.875) -> (93.0508, 15.4399)
  line L662 (93.5623, 17.0142) -> (93.2508, 16.7027)
  line L663 (73.7981, 3.84) -> (73.7981, 3.84)
  line L664 (72.8251, 2.5008) -> (73.2177, 2.7008)
  line L665 (73.7981, 5.94) -> (73.7981, 5.94)
  line L666 (71.0508, 3.4049) -> (71.2508, 3.0123)
  line L667 (73.5292, 6.7677) -> (73.2177, 7.0792)
  line L668 (73.2177, 2.7008) -> (73.5292, 3.0123)
  line L669 (71.0508, 6.3751) -> (70.9819, 5.94)
  line L670 (73.7981, 3.84) -> (73.7981, 5.94)
  line L671 (71.9549, 2.5008) -> (72.39, 2.4319)
  line L672 (73.2177, 7.0792) -> (72.8251, 7.2792)
  line L673 (71.9549, 7.2792) -> (71.5623, 7.0792)
  line L674 (73.7292, 6.3751) -> (73.5292, 6.7677)
  line L675 (71.2508, 6.7677) -> (71.0508, 6.3751)
  line L676 (70.9819, 3.84) -> (71.0508, 3.4049)
  line L677 (73.7981, 5.94) -> (73.7292, 6.3751)
  line L678 (72.39, 7.3481) -> (71.9549, 7.2792)
  line L679 (70.9819, 5.94) -> (70.9819, 3.84)
  line L680 (71.5623, 7.0792) -> (71.2508, 6.7677)
  line L681 (71.2508, 3.0123) -> (71.5623, 2.7008)
  line L682 (72.39, 2.4319) -> (72.8251, 2.5008)
  line L683 (70.9819, 3.84) -> (70.9819, 3.84)
  line L684 (72.8251, 7.2792) -> (72.39, 7.3481)
  line L685 (70.9819, 5.94) -> (70.9819, 5.94)
  line L686 (71.5623, 2.7008) -> (71.9549, 2.5008)
  line L687 (73.5292, 3.0123) -> (73.7292, 3.4049)
  line L688 (73.7292, 3.4049) -> (73.7981, 3.84)
  line L689 (83.6819, 3.84) -> (83.7508, 3.4049)
  line L690 (85.5251, 2.5008) -> (85.9177, 2.7008)
  line L691 (85.09, 7.3481) -> (84.6549, 7.2792)
  line L692 (84.2623, 7.0792) -> (83.9508, 6.7677)
  line L693 (83.6819, 5.94) -> (83.6819, 5.94)
  line L694 (86.4981, 5.94) -> (86.4292, 6.3751)
  line L695 (86.4981, 3.84) -> (86.4981, 5.94)
  line L696 (86.4292, 6.3751) -> (86.2292, 6.7677)
  line L697 (85.5251, 7.2792) -> (85.09, 7.3481)
  line L698 (86.2292, 6.7677) -> (85.9177, 7.0792)
  line L699 (83.6819, 3.84) -> (83.6819, 3.84)
  line L700 (84.6549, 7.2792) -> (84.2623, 7.0792)
  line L701 (85.9177, 2.7008) -> (86.2292, 3.0123)
  line L702 (83.9508, 6.7677) -> (83.7508, 6.3751)
  line L703 (85.9177, 7.0792) -> (85.5251, 7.2792)
  line L704 (83.6819, 5.94) -> (83.6819, 3.84)
  line L705 (84.2623, 2.7008) -> (84.6549, 2.5008)
  line L706 (86.4981, 5.94) -> (86.4981, 5.94)
  line L707 (86.4981, 3.84) -> (86.4981, 3.84)
  line L708 (86.4292, 3.4049) -> (86.4981, 3.84)
  line L709 (85.09, 2.4319) -> (85.5251, 2.5008)
  line L710 (83.7508, 3.4049) -> (83.9508, 3.0123)
  line L711 (86.2292, 3.0123) -> (86.4292, 3.4049)
  line L712 (83.7508, 6.3751) -> (83.6819, 5.94)
  line L713 (84.6549, 2.5008) -> (85.09, 2.4319)
  line L714 (83.9508, 3.0123) -> (84.2623, 2.7008)
  line L715 (3.585, 17.2831) -> (3.1499, 17.2142)
  line L716 (2.4458, 15.0473) -> (2.7573, 14.7358)
  line L717 (5.685, 17.2831) -> (5.685, 17.2831)
  line L718 (2.7573, 17.0142) -> (2.4458, 16.7027)
  line L719 (6.8242, 16.7027) -> (6.5127, 17.0142)
  line L720 (6.5127, 14.7358) -> (6.8242, 15.0473)
  line L721 (5.685, 17.2831) -> (3.585, 17.2831)
  line L722 (2.2458, 15.4399) -> (2.4458, 15.0473)
  line L723 (3.1499, 17.2142) -> (2.7573, 17.0142)
  line L724 (2.2458, 16.3101) -> (2.1769, 15.875)
  line L725 (3.585, 17.2831) -> (3.585, 17.2831)
  line L726 (6.8242, 15.0473) -> (7.0242, 15.4399)
  line L727 (2.4458, 16.7027) -> (2.2458, 16.3101)
  line L728 (7.0242, 16.3101) -> (6.8242, 16.7027)
  line L729 (6.1201, 14.5358) -> (6.5127, 14.7358)
  line L730 (5.685, 14.4669) -> (5.685, 14.4669)
  line L731 (6.5127, 17.0142) -> (6.1201, 17.2142)
  line L732 (7.0242, 15.4399) -> (7.0931, 15.875)
  line L733 (5.685, 14.4669) -> (6.1201, 14.5358)
  line L734 (3.585, 14.4669) -> (5.685, 14.4669)
  line L735 (3.1499, 14.5358) -> (3.585, 14.4669)
  line L736 (2.7573, 14.7358) -> (3.1499, 14.5358)
  line L737 (3.585, 14.4669) -> (3.585, 14.4669)
  line L738 (7.0931, 15.875) -> (7.0242, 16.3101)
  line L739 (6.1201, 17.2142) -> (5.685, 17.2831)
  line L740 (2.1769, 15.875) -> (2.2458, 15.4399)
  line L741 (22.3631, 3.84) -> (22.3631, 5.94)
  line L742 (22.2942, 3.4049) -> (22.3631, 3.84)
  line L743 (20.1273, 2.7008) -> (20.5199, 2.5008)
  line L744 (22.0942, 3.0123) -> (22.2942, 3.4049)
  line L745 (20.1273, 7.0792) -> (19.8158, 6.7677)
  line L746 (22.3631, 3.84) -> (22.3631, 3.84)
  line L747 (20.955, 2.4319) -> (21.3901, 2.5008)
  line L748 (22.3631, 5.94) -> (22.3631, 5.94)
  line L749 (21.7827, 7.0792) -> (21.3901, 7.2792)
  line L750 (21.3901, 2.5008) -> (21.7827, 2.7008)
  line L751 (19.5469, 3.84) -> (19.5469, 3.84)
  line L752 (19.6158, 6.3751) -> (19.5469, 5.94)
  line L753 (19.6158, 3.4049) -> (19.8158, 3.0123)
  line L754 (21.3901, 7.2792) -> (20.955, 7.3481)
  line L755 (19.5469, 3.84) -> (19.6158, 3.4049)
  line L756 (19.5469, 5.94) -> (19.5469, 3.84)
  line L757 (19.8158, 3.0123) -> (20.1273, 2.7008)
  line L758 (22.2942, 6.3751) -> (22.0942, 6.7677)
  line L759 (19.5469, 5.94) -> (19.5469, 5.94)
  line L760 (22.3631, 5.94) -> (22.2942, 6.3751)
  line L761 (19.8158, 6.7677) -> (19.6158, 6.3751)
  line L762 (20.5199, 7.2792) -> (20.1273, 7.0792)
  line L763 (22.0942, 6.7677) -> (21.7827, 7.0792)
  line L764 (20.5199, 2.5008) -> (20.955, 2.4319)
  line L765 (20.955, 7.3481) -> (20.5199, 7.2792)
  line L766 (21.7827, 2.7008) -> (22.0942, 3.0123)
  line L767 (58.2819, 3.84) -> (58.2819, 3.84)
  line L768 (60.5177, 7.0792) -> (60.1251, 7.2792)
  line L769 (60.8292, 3.0123) -> (61.0292, 3.4049)
  line L770 (58.8623, 2.7008) -> (59.2549, 2.5008)
  line L771 (58.2819, 3.84) -> (58.3508, 3.4049)
  line L772 (60.8292, 6.7677) -> (60.5177, 7.0792)
  line L773 (58.5508, 3.0123) -> (58.8623, 2.7008)
  line L774 (58.3508, 3.4049) -> (58.5508, 3.0123)
  line L775 (61.0292, 3.4049) -> (61.0981, 3.84)
  line L776 (60.1251, 7.2792) -> (59.69, 7.3481)
  line L777 (61.0981, 5.94) -> (61.0292, 6.3751)
  line L778 (60.1251, 2.5008) -> (60.5177, 2.7008)
  line L779 (58.2819, 5.94) -> (58.2819, 5.94)
  line L780 (61.0981, 5.94) -> (61.0981, 5.94)
  line L781 (60.5177, 2.7008) -> (60.8292, 3.0123)
  line L782 (61.0981, 3.84) -> (61.0981, 3.84)
  line L783 (61.0981, 3.84) -> (61.0981, 5.94)
  line L784 (58.2819, 5.94) -> (58.2819, 3.84)
  line L785 (58.5508, 6.7677) -> (58.3508, 6.3751)
  line L786 (59.2549, 2.5008) -> (59.69, 2.4319)
  line L787 (58.8623, 7.0792) -> (58.5508, 6.7677)
  line L788 (59.69, 2.4319) -> (60.1251, 2.5008)
  line L789 (58.3508, 6.3751) -> (58.2819, 5.94)
  line L790 (59.69, 7.3481) -> (59.2549, 7.2792)
  line L791 (61.0292, 6.3751) -> (60.8292, 6.7677)
  line L792 (59.2549, 7.2792) -> (58.8623, 7.0792)
  line L793 (32.2469, 5.94) -> (32.2469, 3.84)
  line L794 (32.8273, 2.7008) -> (33.2199, 2.5008)
  line L795 (33.655, 7.3481) -> (33.2199, 7.2792)
  line L796 (32.2469, 3.84) -> (32.3158, 3.4049)
  line L797 (32.5158, 6.7677) -> (32.3158, 6.3751)
  line L798 (34.0901, 7.2792) -> (33.655, 7.3481)
  line L799 (35.0631, 5.94) -> (34.9942, 6.3751)
  line L800 (32.5158, 3.0123) -> (32.8273, 2.7008)
  line L801 (32.3158, 6.3751) -> (32.2469, 5.94)
  line L802 (34.9942, 6.3751) -> (34.7942, 6.7677)
  line L803 (35.0631, 5.94) -> (35.0631, 5.94)
  line L804 (34.7942, 6.7677) -> (34.4827, 7.0792)
  line L805 (32.2469, 5.94) -> (32.2469, 5.94)
  line L806 (34.7942, 3.0123) -> (34.9942, 3.4049)
  line L807 (34.9942, 3.4049) -> (35.0631, 3.84)
  line L808 (35.0631, 3.84) -> (35.0631, 3.84)
  line L809 (32.3158, 3.4049) -> (32.5158, 3.0123)
  line L810 (33.2199, 7.2792) -> (32.8273, 7.0792)
  line L811 (34.0901, 2.5008) -> (34.4827, 2.7008)
  line L812 (32.2469, 3.84) -> (32.2469, 3.84)
  line L813 (34.4827, 7.0792) -> (34.0901, 7.2792)
  line L814 (33.655, 2.4319) -> (34.0901, 2.5008)
  line L815 (34.4827, 2.7008) -> (34.7942, 3.0123)
  line L816 (33.2199, 2.5008) -> (33.655, 2.4319)
  line L817 (35.0631, 3.84) -> (35.0631, 5.94)
  line L818 (32.8273, 7.0792) -> (32.5158, 6.7677)
  line L819 (47.1827, 2.7008) -> (47.4942, 3.0123)
  line L820 (47.1827, 7.0792) -> (46.7901, 7.2792)
  line L821 (47.4942, 3.0123) -> (47.6942, 3.4049)
  line L822 (47.7631, 3.84) -> (47.7631, 5.94)
  line L823 (47.7631, 5.94) -> (47.7631, 5.94)
  line L824 (47.6942, 3.4049) -> (47.7631, 3.84)
  line L825 (45.0158, 6.3751) -> (44.9469, 5.94)
  line L826 (47.6942, 6.3751) -> (47.4942, 6.7677)
  line L827 (45.2158, 6.7677) -> (45.0158, 6.3751)
  line L828 (45.5273, 7.0792) -> (45.2158, 6.7677)
  line L829 (47.7631, 3.84) -> (47.7631, 3.84)
  line L830 (46.355, 2.4319) -> (46.7901, 2.5008)
  line L831 (45.9199, 7.2792) -> (45.5273, 7.0792)
  line L832 (45.5273, 2.7008) -> (45.9199, 2.5008)
  line L833 (47.7631, 5.94) -> (47.6942, 6.3751)
  line L834 (44.9469, 5.94) -> (44.9469, 3.84)
  line L835 (44.9469, 3.84) -> (44.9469, 3.84)
  line L836 (45.2158, 3.0123) -> (45.5273, 2.7008)
  line L837 (44.9469, 5.94) -> (44.9469, 5.94)
  line L838 (46.7901, 2.5008) -> (47.1827, 2.7008)
  line L839 (44.9469, 3.84) -> (45.0158, 3.4049)
  line L840 (45.9199, 2.5008) -> (46.355, 2.4319)
  line L841 (45.0158, 3.4049) -> (45.2158, 3.0123)
  line L842 (47.4942, 6.7677) -> (47.1827, 7.0792)
  line L843 (46.7901, 7.2792) -> (46.355, 7.3481)
  line L844 (46.355, 7.3481) -> (45.9199, 7.2792)
  line L845 (81.3165, 3.84) -> (81.3165, 5.94)
  line L846 (78.8029, 3.34) -> (79.0861, 2.9161)
  line L847 (81.3165, 5.94) -> (81.2171, 6.44)
  line L848 (79.0861, 6.8639) -> (78.8029, 6.44)
  line L849 (80.51, 7.1471) -> (80.01, 7.2465)
  line L850 (81.3165, 3.84) -> (81.3165, 3.84)
  line L851 (80.01, 2.5335) -> (80.51, 2.6329)
  line L852 (80.51, 2.6329) -> (80.9339, 2.9161)
  line L853 (78.8029, 6.44) -> (78.7035, 5.94)
  line L854 (79.51, 7.1471) -> (79.0861, 6.8639)
  line L855 (79.51, 2.6329) -> (80.01, 2.5335)
  line L856 (81.2171, 6.44) -> (80.9339, 6.8639)
  line L857 (81.3165, 5.94) -> (81.3165, 5.94)
  line L858 (80.9339, 2.9161) -> (81.2171, 3.34)
  line L859 (80.01, 7.2465) -> (79.51, 7.1471)
  line L860 (78.7035, 3.84) -> (78.7035, 3.84)
  line L861 (78.7035, 3.84) -> (78.8029, 3.34)
  line L862 (80.9339, 6.8639) -> (80.51, 7.1471)
  line L863 (78.7035, 5.94) -> (78.7035, 3.84)
  line L864 (78.7035, 5.94) -> (78.7035, 5.94)
  line L865 (81.2171, 3.34) -> (81.3165, 3.84)
  line L866 (79.0861, 2.9161) -> (79.51, 2.6329)
  line L867 (16.7989, 2.9161) -> (17.0821, 3.34)
  line L868 (17.0821, 3.34) -> (17.1815, 3.84)
  line L869 (14.6679, 6.44) -> (14.5685, 5.94)
  line L870 (14.5685, 5.94) -> (14.5685, 5.94)
  line L871 (15.875, 7.2465) -> (15.375, 7.1471)
  line L872 (14.5685, 3.84) -> (14.6679, 3.34)
  line L873 (15.375, 7.1471) -> (14.9511, 6.8639)
  line L874 (16.7989, 6.8639) -> (16.375, 7.1471)
  line L875 (15.375, 2.6329) -> (15.875, 2.5335)
  line L876 (17.1815, 5.94) -> (17.1815, 5.94)
  line L877 (14.5685, 5.94) -> (14.5685, 3.84)
  line L878 (16.375, 7.1471) -> (15.875, 7.2465)
  line L879 (17.1815, 3.84) -> (17.1815, 5.94)
  line L880 (14.9511, 6.8639) -> (14.6679, 6.44)
  line L881 (17.0821, 6.44) -> (16.7989, 6.8639)
  line L882 (14.9511, 2.9161) -> (15.375, 2.6329)
  line L883 (15.875, 2.5335) -> (16.375, 2.6329)
  line L884 (17.1815, 5.94) -> (17.0821, 6.44)
  line L885 (14.5685, 3.84) -> (14.5685, 3.84)
  line L886 (14.6679, 3.34) -> (14.9511, 2.9161)
  line L887 (16.375, 2.6329) -> (16.7989, 2.9161)
  line L888 (17.1815, 3.84) -> (17.1815, 3.84)
  line L889 (3.585, 9.4885) -> (5.685, 9.4885)
  line L890 (5.685, 12.1015) -> (5.685, 12.1015)
  line L891 (6.8921, 10.295) -> (6.9915, 10.795)
  line L892 (5.685, 9.4885) -> (5.685, 9.4885)
  line L893 (6.185, 9.5879) -> (6.6089, 9.8711)
  line L894 (3.585, 12.1015) -> (3.585, 12.1015)
  line L895 (3.085, 12.0021) -> (2.6611, 11.7189)
  line L896 (6.6089, 9.8711) -> (6.8921, 10.295)
  line L897 (6.8921, 11.295) -> (6.6089, 11.7189)
  line L898 (2.3779, 10.295) -> (2.6611, 9.8711)
  line L899 (6.6089, 11.7189) -> (6.185, 12.0021)
  line L900 (3.085, 9.5879) -> (3.585, 9.4885)
  line L901 (2.6611, 9.8711) -> (3.085, 9.5879)
  line L902 (2.2785, 10.795) -> (2.3779, 10.295)
  line L903 (6.9915, 10.795) -> (6.8921, 11.295)
  line L904 (2.3779, 11.295) -> (2.2785, 10.795)
  line L905 (3.585, 12.1015) -> (3.085, 12.0021)
  line L906 (6.185, 12.0021) -> (5.685, 12.1015)
  line L907 (2.6611, 11.7189) -> (2.3779, 11.295)
  line L908 (5.685, 9.4885) -> (6.185, 9.5879)
  line L909 (5.685, 12.1015) -> (3.585, 12.1015)
  line L910 (3.585, 9.4885) -> (3.585, 9.4885)
  line L911 (27.2685, 3.84) -> (27.3679, 3.34)
  line L912 (29.8815, 3.84) -> (29.8815, 5.94)
  line L913 (27.6511, 2.9161) -> (28.075, 2.6329)
  line L914 (29.075, 7.1471) -> (28.575, 7.2465)
  line L915 (27.2685, 5.94) -> (27.2685, 3.84)
  line L916 (29.7821, 6.44) -> (29.4989, 6.8639)
  line L917 (28.575, 7.2465) -> (28.075, 7.1471)
  line L918 (29.8815, 3.84) -> (29.8815, 3.84)
  line L919 (27.3679, 3.34) -> (27.6511, 2.9161)
  line L920 (27.2685, 5.94) -> (27.2685, 5.94)
  line L921 (28.075, 7.1471) -> (27.6511, 6.8639)
  line L922 (29.4989, 2.9161) -> (29.7821, 3.34)
  line L923 (27.6511, 6.8639) -> (27.3679, 6.44)
  line L924 (27.3679, 6.44) -> (27.2685, 5.94)
  line L925 (27.2685, 3.84) -> (27.2685, 3.84)
  line L926 (29.075, 2.6329) -> (29.4989, 2.9161)
  line L927 (29.8815, 5.94) -> (29.8815, 5.94)
  line L928 (28.575, 2.5335) -> (29.075, 2.6329)
  line L929 (28.075, 2.6329) -> (28.575, 2.5335)
  line L930 (29.4989, 6.8639) -> (29.075, 7.1471)
  line L931 (29.7821, 3.34) -> (29.8815, 3.84)
  line L932 (29.8815, 5.94) -> (29.7821, 6.44)
  line L933 (52.84, 77.6321) -> (52.4161, 77.3489)
  line L934 (54.5471, 73.825) -> (54.6465, 74.325)
  line L935 (52.84, 73.1179) -> (53.34, 73.0185)
  line L936 (54.2639, 77.3489) -> (53.84, 77.6321)
  line L937 (52.0335, 74.325) -> (52.1329, 73.825)
  line L938 (54.5471, 76.925) -> (54.2639, 77.3489)
  line L939 (53.34, 77.7315) -> (52.84, 77.6321)
  line L940 (54.6465, 74.325) -> (54.6465, 76.425)
  line L941 (54.6465, 76.425) -> (54.6465, 76.425)
  line L942 (54.6465, 76.425) -> (54.5471, 76.925)
  line L943 (53.84, 77.6321) -> (53.34, 77.7315)
  line L944 (52.0335, 76.425) -> (52.0335, 74.325)
  line L945 (52.1329, 76.925) -> (52.0335, 76.425)
  line L946 (54.6465, 74.325) -> (54.6465, 74.325)
  line L947 (53.34, 73.0185) -> (53.84, 73.1179)
  line L948 (54.2639, 73.4011) -> (54.5471, 73.825)
  line L949 (52.1329, 73.825) -> (52.4161, 73.4011)
  line L950 (52.4161, 73.4011) -> (52.84, 73.1179)
  line L951 (52.0335, 76.425) -> (52.0335, 76.425)
  line L952 (52.4161, 77.3489) -> (52.1329, 76.925)
  line L953 (52.0335, 74.325) -> (52.0335, 74.325)
  line L954 (53.84, 73.1179) -> (54.2639, 73.4011)
  line L955 (41.275, 2.5335) -> (41.775, 2.6329)
  line L956 (39.9685, 5.94) -> (39.9685, 5.94)
  line L957 (39.9685, 3.84) -> (40.0679, 3.34)
  line L958 (42.1989, 2.9161) -> (42.4821, 3.34)
  line L959 (40.775, 2.6329) -> (41.275, 2.5335)
  line L960 (42.4821, 3.34) -> (42.5815, 3.84)
  line L961 (40.0679, 6.44) -> (39.9685, 5.94)
  line L962 (40.775, 7.1471) -> (40.3511, 6.8639)
  line L963 (40.3511, 2.9161) -> (40.775, 2.6329)
  line L964 (42.5815, 3.84) -> (42.5815, 3.84)
  line L965 (41.775, 2.6329) -> (42.1989, 2.9161)
  line L966 (42.5815, 5.94) -> (42.4821, 6.44)
  line L967 (42.4821, 6.44) -> (42.1989, 6.8639)
  line L968 (39.9685, 5.94) -> (39.9685, 3.84)
  line L969 (42.1989, 6.8639) -> (41.775, 7.1471)
  line L970 (40.0679, 3.34) -> (40.3511, 2.9161)
  line L971 (42.5815, 3.84) -> (42.5815, 5.94)
  line L972 (41.275, 7.2465) -> (40.775, 7.1471)
  line L973 (42.5815, 5.94) -> (42.5815, 5.94)
  line L974 (39.9685, 3.84) -> (39.9685, 3.84)
  line L975 (41.775, 7.1471) -> (41.275, 7.2465)
  line L976 (40.3511, 6.8639) -> (40.0679, 6.44)
  line L977 (54.11, 2.6329) -> (54.61, 2.5335)
  line L978 (55.9165, 3.84) -> (55.9165, 3.84)
  line L979 (53.6861, 2.9161) -> (54.11, 2.6329)
  line L980 (55.9165, 5.94) -> (55.8171, 6.44)
  line L981 (54.61, 2.5335) -> (55.11, 2.6329)
  line L982 (54.11, 7.1471) -> (53.6861, 6.8639)
  line L983 (55.8171, 3.34) -> (55.9165, 3.84)